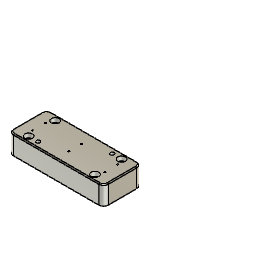
CAD_File 9 (Autodesk Fusion 360 design; units mm, degrees)
Autodesk Fusion 360 part; units mm, degrees
note: some values were not read from the file. Chosen so that the rebuilt part matches the saved one: a direction; where a step ends. Set by a fixed rule: which sketch regions a step uses.
sketch "Sketch2" plane through (0, 0, 0) normal (0, 0, 1) x (1, 0, 0)
  line L0 (124, -242) -> (124, -20)
  line L1 (124, -20) -> (-124, -20)
  circle A0 centre (-115, -40) radius 5.5
  circle A1 centre (-115, -137) radius 5.5
  line L2 (-124, -20) -> (-124, -242)
  line L3 (-124, -242) -> (124, -242)
  circle A2 centre (115, -137) radius 5.5
  circle A3 centre (115, -40) radius 5.5
  circle A4 centre (0, -187) radius 14
  circle A5 centre (15, -202) radius 1.1354
  circle A6 centre (-15, -202) radius 1.1354
  circle A7 centre (15, -172) radius 1.1354
  circle A8 centre (-15, -172) radius 1.1354
  line L4 (45, -101.5) -> (-45, -101.5)
  line L5 (-50, -96.5) -> (-50, -66.5)
  line L6 (50, -66.5) -> (50, -96.5)
  line L7 (50, -101.5) -> (-50, -61.5) construction
  line L8 (-50, -101.5) -> (50, -61.5) construction
  arc A9 (-45, -61.5) -> (-50, -66.5) centre (-45, -66.5) ccw
  arc A10 (-50, -96.5) -> (-45, -101.5) centre (-45, -96.5) ccw
  arc A11 (45, -101.5) -> (50, -96.5) centre (45, -96.5) ccw
  arc A12 (50, -66.5) -> (45, -61.5) centre (45, -66.5) ccw
  line L9 (45, -61.5) -> (-45, -61.5)
  circle A13 centre (-115, -234) radius 5.5
  circle A14 centre (115, -234) radius 5.5
  point P0 (0, -81.5)
  dimension "d287" = 100
  dimension "d288" = 40
  dimension "d289" = 5
  constraint horizontal L4
  constraint perpendicular L4 L5
  constraint parallel L5 L6
  constraint coincident L7 P0
  constraint coincident L8 P0
  constraint coincident L7.end L5
  constraint tangent L5 A9
  constraint coincident L8.start L5
  constraint coincident L8.start L4
  constraint tangent L5 A10
  constraint tangent L4 A10
  constraint equal A9 A10
  constraint coincident L7.start L4
  constraint coincident L7.start L6
  constraint tangent L4 A11
  constraint tangent L6 A11
  constraint equal A9 A11
  constraint coincident L8.end L6
  constraint tangent L6 A12
  constraint equal A9 A12
  constraint tangent A9 L9
  measures "d287" distance of L7.end L8.end
  measures "d288" distance of L8.start L7.end
  measures "d289" radius of A9
extrude "Extrude1" add sketch "Sketch2" along normal blind 8 contours L4 L5 L6 A9 A10 A11 A12 L9
sketch "Sketch4" plane through (0, 0, 0) normal (0, 0, -1) x (1, 0, 0)
  arc A0 (45, 61.5) -> (50, 66.5) centre (45, 66.5) ccw
  line L0 (50, 66.5) -> (50, 96.5)
  arc A1 (50, 96.5) -> (45, 101.5) centre (45, 96.5) ccw
  line L1 (45, 101.5) -> (-45, 101.5)
  arc A2 (-45, 101.5) -> (-50, 96.5) centre (-45, 96.5) ccw
  line L2 (-50, 96.5) -> (-50, 66.5)
  arc A3 (-50, 66.5) -> (-45, 61.5) centre (-45, 66.5) ccw
  line L3 (-45, 61.5) -> (45, 61.5)
  circle A4 centre (-38, -74.8) radius 1.75
  circle A5 centre (-38, -88.2) radius 1.75
  circle A6 centre (0, -74.8) radius 1.75
  circle A7 centre (0, -88.2) radius 1.75
  circle A8 centre (38, -74.8) radius 1.75
  circle A9 centre (38, -88.2) radius 1.75
  dimension "d320" = 3.5
  dimension "d321" = 3.5
  dimension "d322" = 3.5
  dimension "d323" = 3.5
  dimension "d324" = 3.5
  dimension "d325" = 3.5
  measures "d320" diameter of A4
  measures "d321" diameter of A5
  measures "d322" diameter of A6
  measures "d323" diameter of A7
  measures "d324" diameter of A8
  measures "d325" diameter of A9
extrude "Extrude5" cut sketch "Sketch4" against normal blind 5 contours A4 | A5 | A6 | A7 | A8 | A9
chamfer "Chamfer1" distance 1 angle 45 8 edges at (50, -81.5, 8) (48.5355, -62.9645, 8) (0, -61.5, 8) (-48.5355, -62.9645, 8) (-50, -81.5, 8) (-48.5355, -100.0355, 8) (0, -101.5, 8) (48.5355, -100.0355, 8)
move_face "OffsetFaces1" offset 12 1 faces at (15, -88.1667, 0)
sketch "Sketch5" plane through (0, 0, 8) normal (0, 0, 1) x (-1, 0, 0)
  circle A0 centre (38, 74.8) radius 0.8
  circle A1 centre (-38, 74.8) radius 0.8
  circle A2 centre (0, 74.8) radius 0.8
  circle A3 centre (38, 88.2) radius 0.8
  circle A4 centre (-38, 88.2) radius 0.8
  circle A5 centre (0, 88.2) radius 0.8
  circle A6 centre (35, 67.5) radius 2.1
  circle A7 centre (-25, 67.5) radius 2
  circle A8 centre (-35, 95.5) radius 2.1
  circle A9 centre (35, 95.5) radius 2.1
  circle A10 centre (-35, 67.5) radius 2.1
  circle A11 centre (25, 95.5) radius 2
  line L0 (-49, 96.5) -> (-49, 66.5)
  arc A12 (-49, 66.5) -> (-45, 62.5) centre (-45, 66.5) ccw
  line L1 (-45, 62.5) -> (45, 62.5)
  arc A13 (45, 62.5) -> (49, 66.5) centre (45, 66.5) ccw
  line L2 (49, 66.5) -> (49, 96.5)
  arc A14 (49, 96.5) -> (45, 100.5) centre (45, 96.5) ccw
  line L3 (45, 100.5) -> (-45, 100.5)
  arc A15 (-45, 100.5) -> (-49, 96.5) centre (-45, 96.5) ccw
  circle A16 centre (35, 67.5) radius 4
  circle A17 centre (35, 95.5) radius 4
  circle A18 centre (-35, 67.5) radius 4
  circle A19 centre (-35, 95.5) radius 4
  line L4 (50, 66.5) -> (50, 96.5)
  line L5 (-45, 61.5) -> (45, 61.5)
  line L6 (45, 101.5) -> (-45, 101.5)
  line L7 (0, 55) -> (0, 110) construction
  line L8 (55, 81.5) -> (-56, 81.5) construction
  dimension "d494" = 4.2
  dimension "d495" = 4.2
  dimension "d496" = 4.2
  dimension "d497" = 4.2
  dimension "d498" = 4
  dimension "d499" = 4
  dimension "d500" = 8
  dimension "d501" = 8
  dimension "d502" = 8
  dimension "d503" = 8
  dimension "d504" = 15
  dimension "d505" = 6
  dimension "d506" = 6
  dimension "d507" = 6
  dimension "d508" = 20
  constraint concentric A6 A16
  constraint concentric A9 A17
  constraint concentric A10 A18
  constraint concentric A8 A19
  constraint perpendicular L3 L7
  constraint perpendicular L0 L8
  constraint symmetric A16 A18 L7
  constraint symmetric A16 A17 L8
  constraint symmetric A18 A19 L8
  measures "d494" diameter of A6
  measures "d495" diameter of A9
  measures "d496" diameter of A8
  measures "d497" diameter of A10
  measures "d498" diameter of A7
  measures "d499" diameter of A11
  measures "d500" diameter of A16
  measures "d501" diameter of A17
  measures "d502" diameter of A18
  measures "d503" diameter of A19
  measures "d504" distance of A6.centre L4
  measures "d505" distance of A6.centre L5
  measures "d506" distance of A11.centre L6
  measures "d507" distance of A7.centre L5
  measures "d508" distance of L5 L8
extrude "Extrude6" cut sketch "Sketch5" along normal up to far side of body 1 contours A0 | A1 | A2 | A3 | A4 | A5 | A6 | A7 | A8 | A9 | A10 | A11
extrude "Extrude7" cut sketch "Sketch5" against normal blind 4.5 contours A16 | A17 | A18 | A19
sketch "Sketch6" plane through (0, 0, -12) normal (0, 0, -1) x (1, 0, 0)
  circle A0 centre (38, 74.8) radius 0.8
  circle A1 centre (0, 74.8) radius 0.8
  circle A2 centre (-35, 95.5) radius 2.1
  circle A3 centre (-25, 95.5) radius 2
  circle A4 centre (0, 88.2) radius 0.8
  circle A5 centre (38, 88.2) radius 0.8
  circle A6 centre (25, 67.5) radius 2
  circle A7 centre (-38, 74.8) radius 0.8
  circle A8 centre (-35, 67.5) radius 2.1
  circle A9 centre (-38, 88.2) radius 0.8
  circle A10 centre (35, 67.5) radius 2.1
  circle A11 centre (35, 95.5) radius 2.1
  arc A12 (45, 61.5) -> (50, 66.5) centre (45, 66.5) ccw
  line L0 (50, 66.5) -> (50, 96.5)
  arc A13 (50, 96.5) -> (45, 101.5) centre (45, 96.5) ccw
  line L1 (45, 101.5) -> (-45, 101.5)
  arc A14 (-45, 101.5) -> (-50, 96.5) centre (-45, 96.5) ccw
  line L2 (-50, 96.5) -> (-50, 66.5)
  arc A15 (-50, 66.5) -> (-45, 61.5) centre (-45, 66.5) ccw
  line L3 (-45, 61.5) -> (45, 61.5)
  circle A16 centre (-38, 88.2) radius 1.75
  circle A17 centre (-38, 74.8) radius 1.75
  circle A18 centre (0, 88.2) radius 1.75
  circle A19 centre (0, 74.8) radius 1.75
  circle A20 centre (38, 88.2) radius 1.75
  circle A21 centre (38, 74.8) radius 1.75
  dimension "d737" = 3.5
  dimension "d738" = 3.5
  dimension "d739" = 3.5
  dimension "d740" = 3.5
  dimension "d741" = 3.5
  dimension "d742" = 3.5
  constraint concentric A9 A16
  constraint concentric A7 A17
  constraint concentric A4 A18
  constraint concentric A1 A19
  constraint concentric A5 A20
  constraint concentric A0 A21
  measures "d737" diameter of A16
  measures "d738" diameter of A17
  measures "d739" diameter of A18
  measures "d740" diameter of A19
  measures "d741" diameter of A20
  measures "d742" diameter of A21
extrude "Extrude8" cut sketch "Sketch6" against normal blind 3 contours A16 | A17 | A18 | A19 | A20 | A21
